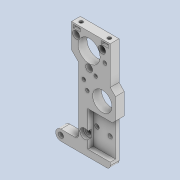
# Autodesk Inventor part: PartA_3D
Saved by Autodesk Inventor 2020.4 (Build 244396000, 396)
## iProperties
Created: 2020-12-02
Part Number: PartA_3D
Material: Generic
Document SubType Name: Modeling
Designer: Acer
Density: 1 g/cm^3
Appearance: Default
Author: Acer
Autodesk Inventor part; units mm, degrees
ref_plane "YZ Plane" through (0, 0, 0) normal (1, 0, 0) x (0, 1, 0)
ref_plane "XZ Plane" through (0, 0, 0) normal (0, 1, 0) x (-1, 0, 0)
ref_plane "XY Plane" through (0, 0, 0) normal (0, 0, 1) x (1, 0, 0)
sketch "Sketch1" plane through (0, 0, 0) normal (0, 0, 1) x (1, 0, 0)
  circle A0 centre (0, 0) radius 1.5
  circle A1 centre (0, 0) radius 3
  line L0 (0, 3) -> (28, 3)
  line L1 (28, 3) -> (28, -3)
  line L2 (28, -3) -> (0, -3)
  line L3 (0, -3) -> (0, 3)
  line L4 (28, 3) -> (10, 3)
  line L5 (10, 3) -> (10, 59)
  line L6 (10, 59) -> (28, 59)
  line L7 (28, 59) -> (28, 3)
  circle A2 centre (23.5, 28.5) radius 5.5
  circle A3 centre (15.9973, 49.5) radius 6.25
  line L8 (23.5, 28.5) -> (15.9973, 49.5) construction
  line L9 (23.5, 28.5) -> (10, 28.5) construction
  circle A4 centre (15.9973, 41) radius 1.05
  circle A5 centre (23.3585, 53.75) radius 1.05
  circle A6 centre (8.6361, 53.75) radius 1.05
  line L10 (10, 59) -> (6, 59)
  line L11 (6, 59) -> (6, 45)
  line L12 (6, 45) -> (10, 45)
  line L13 (10, 45) -> (10, 59)
  line L14 (6, 45) -> (10, 41)
  line L15 (6, 45) -> (11.6569, 45) construction
  line L16 (28, 34.5) -> (31, 34.5)
  line L17 (31, 34.5) -> (31, 22.5)
  line L18 (31, 22.5) -> (28, 22.5)
  line L19 (28, 22.5) -> (28, 34.5)
  line L20 (31, 34.5) -> (28, 37.5)
  line L21 (31, 34.5) -> (35.2426, 34.5) construction
  line L22 (31, 22.5) -> (28, 19.5)
  line L23 (31, 22.5) -> (35.2426, 22.5) construction
  circle A7 centre (13.5, 7.5) radius 1.5
  circle A8 centre (17.5, 11.5) radius 1.25
  circle A9 centre (25, 10.5) radius 1.25
  line L24 (15.9973, 49.5) -> (6, 49.5) construction
  line L25 (15.9973, 41) -> (15.9973, 49.5) construction
  circle A10 centre (19.7487, 39) radius 1
  circle A11 centre (15, 29.5) radius 1.05
  circle A12 centre (13, 34) radius 1.05
  circle A13 centre (25, 48) radius 1.05
  line L26 (10, 27) -> (28, 27) construction
  line L27 (28, 27) -> (28, 51) construction
  line L28 (28, 51) -> (10, 51) construction
  line L29 (10, 51) -> (10, 27) construction
  line L30 (11.7876, 31.9) -> (10.5751, 34) construction
  line L31 (10.5751, 34) -> (11.7876, 36.1) construction
  line L32 (11.7876, 36.1) -> (14.2124, 36.1) construction
  line L33 (14.2124, 36.1) -> (15.4249, 34) construction
  line L34 (15.4249, 34) -> (14.2124, 31.9) construction
  line L35 (14.2124, 31.9) -> (11.7876, 31.9) construction
  line L36 (13.7876, 27.4) -> (12.5751, 29.5) construction
  line L37 (12.5751, 29.5) -> (13.7876, 31.6) construction
  line L38 (13.7876, 31.6) -> (16.2124, 31.6) construction
  line L39 (16.2124, 31.6) -> (17.4249, 29.5) construction
  line L40 (17.4249, 29.5) -> (16.2124, 27.4) construction
  line L41 (16.2124, 27.4) -> (13.7876, 27.4) construction
  dimension "d0" = 3
  dimension "d1" = 6
  dimension "d2" = 28
  dimension "d3" = 6
  dimension "d4" = 0
  dimension "d5" = 3
  dimension "d6" = 18
  dimension "d7" = 56
  dimension "d8" = 11
  dimension "d9" = 4.5
  dimension "d10" = 25.5
  dimension "d11" = 12.5
  dimension "d12" = 22.3
  dimension "d14" = 2.1
  dimension "d17" = 9.5
  dimension "d20" = 360
  dimension "d22" = 4
  dimension "d23" = 14
  dimension "d24" = 45
  dimension "d25" = 3
  dimension "d26" = 12
  dimension "d27" = 6
  dimension "d28" = 135
  dimension "d29" = 135
  dimension "d32" = 3
  dimension "d33" = 10.5
  dimension "d34" = 3.5
  dimension "d35" = 2.5
  dimension "d36" = 14.5
  dimension "d37" = 7.5
  dimension "d38" = 2.5
  dimension "d39" = 15
  dimension "d40" = 13.5
  dimension "d60" = 8.5
  dimension "d61" = 270
  dimension "d82" = 2
  dimension "d83" = 11.15
  dimension "d84" = 2.1
  dimension "d85" = 2.1
  dimension "d86" = 2.1
  dimension "d87" = 5
  dimension "d88" = 3
  dimension "d89" = 25
  dimension "d90" = 29.5
  dimension "d91" = 3
  dimension "d92" = 11
  dimension "d93" = 24
  dimension "d94" = 8
  dimension "d101" = 2.1
  dimension "d102" = 2.1
  constraints: 84 end point, 14 centre point, 11 horizontal, 10 parallel, 8 point on line, 6 perpendicular, 4 coincident, 3 equal length, 1 midpoint, 33 other
  measures "d0" diameter of A0
  measures "d1" diameter of A1
  measures "d2" distance of L1.end L2.end
  measures "d3" distance of L0.end L1.end
  measures "d4" distance from line of point (0, 0) L3
  measures "d5" distance from line of L0 point (0, 0)
  measures "d6" distance of L5.end L6.end
  measures "d7" distance of L4.end L5.end
  measures "d8" diameter of A2
  measures "d9" distance from line of L7 L8.start
  measures "d10" distance from line of L8.start L0
  measures "d11" diameter of A3
  measures "d12" distance of L8.start L8.end
  measures "d14" diameter of A4
  measures "d17" distance from line of L6 L8.end
  measures "d22" distance of L12.end L11.end
  measures "d23" distance of L11.end L10.end
  measures "d24" angle of L14 L15
  measures "d25" distance of L17.end L18.end
  measures "d26" distance of L16.end L17.end
  measures "d27" distance from line of L16 L8.start
  measures "d28" angle of L21 L20
  measures "d29" angle of L22 L23
  measures "d32" diameter of A7
  measures "d33" distance from line of L2 A7.centre
  measures "d34" distance from line of L5 A7.centre
  measures "d35" diameter of A8
  measures "d36" distance from line of A8.centre L2
  measures "d37" distance from line of L5 A8.centre
  measures "d38" diameter of A9
  measures "d39" distance from line of A9.centre L5
  measures "d40" distance from line of L2 A9.centre
  measures "d60" distance of L25.start L8.end
  measures "d82" diameter of A10
  measures "d83" distance of A10.centre L8.start
  measures "d84" diameter of A11
  measures "d85" diameter of A12
  measures "d86" diameter of A13
  measures "d87" distance from line of L5 A11.centre
  measures "d88" distance from line of L5 A12.centre
  measures "d89" distance from line of L6 A12.centre
  measures "d90" distance from line of L6 A11.centre
  measures "d91" distance from line of L7 A13.centre
  measures "d92" distance from line of L6 A13.centre
  measures "d93" distance between parallel lines of L28 L26
  measures "d94" distance between parallel lines of L6 L28
  measures "d101" distance from line of A12.centre L35
  measures "d102" distance from line of A11.centre L41
extrude "Extrusion1" add sketch "Sketch1" along normal blind 5 contours A0 L3 A1 | A0 L3 A1 | L0 L1 L2 A1 | L5 A3 L6 L7 A2 L0 | L14 L12 L5 | L7 L18 L22 | L12 L11 L10 L5 A3 | L7 A2 L16 L17 L18 | L16 L7 L20
fillet "Fillet1" radius 2 1 edges at (28, -3, 2.5)
fillet "Fillet2" radius 2 1 edges at (10, 3, 2.5)
sketch "Sketch2" plane through (0, 0, 5) normal (0, 0, 1) x (1, 0, 0)
  line L0 (28, -1) -> (28, 19.5) projected
  line L1 (0, -3) -> (26, -3) projected
  line L2 (28, -1) -> (28, 19.5) projected
  line L3 (28, 20.75) -> (15.25, 20.75)
  line L4 (15.25, 20.75) -> (15.25, 0.75)
  line L5 (15.25, 0.75) -> (28, 0.75)
  line L6 (28, 0.75) -> (28, 20.75)
  line L7 (28, 19.5) -> (31, 22.5) projected
  line L8 (28, 20.75) -> (29.25, 20.75)
  line L9 (28, 19.5) -> (31, 22.5) projected
  line L10 (26.75, 20.75) -> (26.75, 0.75)
  point P0 (0, 0)
  point P1 (28, 19.5)
  point P2 (28, 19.5)
  dimension "d43" = 12.75
  dimension "d44" = 20
  dimension "d45" = 23.75
  constraints: 12 end point, 4 point on line, 2 horizontal, 2 parallel, 2 perpendicular
  measures "d43" distance of L5.end L4.end
  measures "d44" distance of L4.end L3.end
  measures "d45" distance between parallel lines of L1 L3
extrude "Extrusion2" cut sketch "Sketch2" against normal blind 3
sketch "Sketch3" plane through (6, 59, 0) normal (0, 1, 0) x (1, 0, 0)
  circle A0 centre (3, -2.5) radius 1
  line L0 (22, 0) -> (0, 0) projected
  line L1 (0, 0) -> (0, -5) projected
  line L2 (22, -5) -> (0, -5) projected
  line L3 (22, 0) -> (22, -5) projected
  circle A1 centre (19, -2.5) radius 1
  dimension "d48" = 2
  dimension "d49" = 2
  dimension "d50" = 2.5
  dimension "d51" = 2.5
  dimension "d52" = 3
  dimension "d53" = 3
  constraints: 2 centre point
  measures "d48" diameter of A0
  measures "d49" diameter of A1
  measures "d50" distance from line of L0 A0.centre
  measures "d51" distance from line of L0 A1.centre
  measures "d52" distance from line of A1.centre L3
  measures "d53" distance from line of L1 A0.centre
extrude "Extrusion3" cut sketch "Sketch3" against normal blind 3 contours A0 | A1
thread "Thread1" size "M2x0.4" class "6H" standard "ANSI Metric M Profile" length 7
thread "Thread2" size "M2x0.4" class "6H" standard "ANSI Metric M Profile" length 7
sketch "Sketch5" plane through (0, 0, 5) normal (0, 0, 1) x (1, 0, 0)
  circle A0 centre (15.9973, 41) radius 1.05 projected
  circle A1 centre (8.6361, 53.75) radius 1.05 projected
  circle A2 centre (23.3585, 53.75) radius 1.05 projected
  circle A3 centre (15.9973, 41) radius 2
  circle A4 centre (8.6361, 53.75) radius 2
  circle A5 centre (23.3585, 53.75) radius 2
  point P0 (0, 0)
  dimension "d62" = 4
  dimension "d63" = 4
  dimension "d64" = 4
  constraints: 3 centre point, 3 coincident
  measures "d62" diameter of A3
  measures "d63" diameter of A4
  measures "d64" diameter of A5
extrude "Extrusion4" cut sketch "Sketch5" against normal blind 3 contours A0 | A1 | A2 | A3 | A4 | A5
sketch "Sketch7" plane through (0, 0, 5) normal (0, 0, 1) x (1, 0, 0)
  circle A0 centre (13.5, 7.5) radius 1.5 projected
  circle A1 centre (13.5, 7.5) radius 2.75
  point P0 (0, 0)
  dimension "d67" = 5.5
  constraints: 1 centre point, 1 coincident
  measures "d67" diameter of A1
extrude "Extrusion5" cut sketch "Sketch7" against normal blind 2 contours A0 | A1
sketch "Sketch8" plane through (0, 0, 5) normal (0, 0, 1) x (1, 0, 0)
  line L0 (10, 59) -> (10, 56) projected
  line L1 (8, 59) -> (8, 56) projected
  circle A0 centre (23.3585, 53.75) radius 2 projected
  circle A1 centre (8.6361, 53.75) radius 2 projected
  circle A2 centre (15.9973, 41) radius 2 projected
  circle A3 centre (23.5, 28.5) radius 5.5 projected
  circle A4 centre (15.9973, 49.5) radius 6.25 projected
  arc A5 (15.25, 9.6213) -> (15.25, 5.3787) centre (13.5, 7.5) ccw projected
  line L2 (15.25, 9.6213) -> (15.25, 20.75) projected
  line L3 (15.25, 20.75) -> (29.25, 20.75) projected
  line L4 (29.25, 20.75) -> (31, 22.5) projected
  line L5 (31, 22.5) -> (31, 34.5) projected
  line L6 (31, 34.5) -> (28, 37.5) projected
  line L7 (28, 37.5) -> (28, 59) projected
  line L8 (28, 59) -> (6, 59) projected
  line L9 (6, 59) -> (6, 45) projected
  line L10 (6, 45) -> (10, 41) projected
  line L11 (10, 41) -> (10, 5) projected
  line L12 (24, 59) -> (24, 56) projected
  line L13 (26, 59) -> (26, 56) projected
  line L14 (7, 56.275) -> (11, 56.275)
  line L15 (11, 56.275) -> (11, 58.125)
  line L16 (11, 58.125) -> (7, 58.125)
  line L17 (7, 58.125) -> (7, 56.275)
  line L18 (7, 56.275) -> (11, 58.125) construction
  line L19 (11, 56.275) -> (7, 58.125) construction
  line L20 (23, 58.125) -> (27, 58.125)
  line L21 (27, 58.125) -> (27, 56.275)
  line L22 (27, 56.275) -> (23, 56.275)
  line L23 (23, 56.275) -> (23, 58.125)
  line L24 (23, 58.125) -> (27, 56.275) construction
  line L25 (27, 58.125) -> (23, 56.275) construction
  arc A6 (8, 3) -> (10, 5) centre (8, 5) ccw projected
  line L26 (8, 3) -> (0, 3) projected
  arc A7 (0, 3) -> (0, -3) centre (0, 0) ccw projected
  line L27 (0, -3) -> (26, -3) projected
  arc A8 (26, -3) -> (28, -1) centre (26, -1) ccw projected
  line L28 (28, -1) -> (28, 0.75) projected
  line L29 (28, 0.75) -> (15.25, 0.75) projected
  line L30 (15.25, 0.75) -> (15.25, 5.3787) projected
  point P0 (9, 57.2)
  point P1 (25, 57.2)
  dimension "d70" = 4
  dimension "d71" = 1.85
  dimension "d72" = 4
  dimension "d73" = 1.85
  dimension "d74" = 1
  dimension "d75" = 1.8
  dimension "d76" = 1.8
  dimension "d77" = 1
  constraints: 24 end point, 4 midpoint, 4 parallel, 2 horizontal, 2 perpendicular
  measures "d70" distance of L16.end L15.end
  measures "d71" distance of L15.end L14.end
  measures "d72" distance of L21.end L22.end
  measures "d73" distance of L20.end L21.end
  measures "d74" distance from line of point (9, 57.2) L0
  measures "d75" distance from line of L8 point (9, 57.2)
  measures "d76" distance from line of L8 point (25, 57.2)
  measures "d77" distance from line of point (25, 57.2) L13
extrude "Extrusion6" cut sketch "Sketch8" against normal up to surface (5 mm away) contours L16 L15 L14 L0 | L0 L14 L1 L16 | L1 L14 L17 L16 | L20 L13 L22 L12 | L12 L22 L23 L20 | L20 L21 L22 L13
sketch "Sketch10" plane through (0, 0, 0) normal (0, 0, -1) x (-1, 0, 0)
  circle A0 centre (-25, 48) radius 1.05 projected
  circle A1 centre (-13, 34) radius 1.05 projected
  circle A2 centre (-15, 29.5) radius 1.05 projected
  line L0 (-26.2124, 45.9) -> (-27.4249, 48)
  line L1 (-27.4249, 48) -> (-26.2124, 50.1)
  line L2 (-26.2124, 50.1) -> (-23.7876, 50.1)
  line L3 (-23.7876, 50.1) -> (-22.5751, 48)
  line L4 (-22.5751, 48) -> (-23.7876, 45.9)
  line L5 (-23.7876, 45.9) -> (-26.2124, 45.9)
  line L6 (-16.2124, 27.4) -> (-17.4249, 29.5)
  line L7 (-17.4249, 29.5) -> (-16.2124, 31.6)
  line L8 (-16.2124, 31.6) -> (-13.7876, 31.6)
  line L9 (-13.7876, 31.6) -> (-12.5751, 29.5)
  line L10 (-12.5751, 29.5) -> (-13.7876, 27.4)
  line L11 (-13.7876, 27.4) -> (-16.2124, 27.4)
  line L12 (-14.2124, 31.9) -> (-15.4249, 34)
  line L13 (-15.4249, 34) -> (-14.2124, 36.1)
  line L14 (-14.2124, 36.1) -> (-11.7876, 36.1)
  line L15 (-11.7876, 36.1) -> (-10.5751, 34)
  line L16 (-10.5751, 34) -> (-11.7876, 31.9)
  line L17 (-11.7876, 31.9) -> (-14.2124, 31.9)
  point P0 (0, 0)
  point P1 (-13.9053, 32.1)
  point P2 (-12.0947, 30.9)
  dimension "d95" = 2.1
  dimension "d96" = 2.1
  dimension "d98" = 2.1
  constraints: 36 end point, 4 coincident, 3 horizontal, 39 other
  measures "d95" distance from line of A0.centre L5
  measures "d96" distance from line of A2.centre L11
  measures "d98" distance from line of A1.centre L17
extrude "Extrusion7" cut sketch "Sketch10" against normal blind 1.8 contours A1 | A2 | L0 L1 L2 L3 L4 L5 | L6 L7 L8 L9 L10 L11 | L12 L13 L14 L15 L16 L17
body "Solid1"
